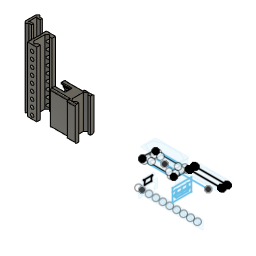
2022_09_14_ThetaSStereoOnPicaTinny v2 (Autodesk Fusion 360 design; units mm, degrees)
Autodesk Fusion 360 part; units mm, degrees
sketch "Sketch1" plane through (0, 0, 0) normal (0, 0, 1) x (1, 0, 0)
  line L0 (9.6991, 0) -> (35.3009, 0)
  line L1 (45, 5.4642) -> (45, 13.4642)
  line L2 (35.2828, 19) -> (9.7172, 19)
  line L3 (0, 13.4642) -> (0, 5.4642)
  line L4 (0, 9.4642) -> (4, 9.4642) construction
  line L5 (4, 9.4642) -> (4, 16.4642) construction
  line L6 (4, 9.4642) -> (4, 2.4642) construction
  line L7 (45, 9.4642) -> (41, 9.4642) construction
  line L8 (41, 9.4642) -> (41, 16.4642) construction
  line L9 (41, 9.4642) -> (41, 2.4642) construction
  line L10 (3.5218, 16.4642) -> (3, 16.4642)
  line L11 (3.3009, 2.4642) -> (3, 2.4642)
  line L12 (41.6991, 2.4642) -> (42, 2.4642)
  line L13 (41.7172, 16.4642) -> (42, 16.4642)
  line L14 (4, 9.4642) -> (9, 9.4642) construction
  line L15 (41, 9.4642) -> (36, 9.4642) construction
  line L16 (36, 9.4642) -> (36, 19) construction
  line L17 (36, 9.4642) -> (36, 0) construction
  line L18 (9, 9.4642) -> (9, 0) construction
  line L19 (9, 9.4642) -> (9, 19) construction
  line L20 (4.4265, 16.6805) -> (8.3603, 18.6756)
  line L21 (36.6397, 18.6756) -> (40.3603, 16.7887)
  line L22 (40.3729, 2.1552) -> (36.6271, 0.3091)
  line L23 (8.3729, 0.3091) -> (4.6271, 2.1552)
  line L24 (0, -1.771) -> (45, -1.771)
  line L25 (47, 0.229) -> (47, 18.6995)
  line L26 (45, 20.6995) -> (0, 20.6995)
  line L27 (-2, 18.6995) -> (-2, 0.229)
  arc A0 (47, 18.6995) -> (45, 20.6995) centre (45, 18.6995) ccw
  arc A1 (45, -1.771) -> (47, 0.229) centre (45, 0.229) ccw
  arc A2 (-2, 0.229) -> (0, -1.771) centre (0, 0.229) ccw
  arc A3 (0, 20.6995) -> (-2, 18.6995) centre (0, 18.6995) ccw
  arc A4 (3.5218, 16.4642) -> (4.4265, 16.6805) centre (3.5218, 18.4642) ccw
  arc A5 (4.6271, 2.1552) -> (3.3009, 2.4642) centre (3.3009, -0.5358) ccw
  arc A6 (40.3603, 16.7887) -> (41.7172, 16.4642) centre (41.7172, 19.4642) ccw
  arc A7 (41.6991, 2.4642) -> (40.3729, 2.1552) centre (41.6991, -0.5358) ccw
  arc A8 (45, 13.4642) -> (42, 16.4642) centre (42, 13.4642) ccw
  arc A9 (42, 2.4642) -> (45, 5.4642) centre (42, 5.4642) ccw
  arc A10 (0, 5.4642) -> (3, 2.4642) centre (3, 5.4642) ccw
  arc A11 (3, 16.4642) -> (0, 13.4642) centre (3, 13.4642) ccw
  arc A12 (9.7172, 19) -> (8.3603, 18.6756) centre (9.7172, 16) ccw
  arc A13 (36.6397, 18.6756) -> (35.2828, 19) centre (35.2828, 16) ccw
  arc A14 (35.3009, 0) -> (36.6271, 0.3091) centre (35.3009, 3) ccw
  arc A15 (8.3729, 0.3091) -> (9.6991, 0) centre (9.6991, 3) ccw
  line L28 (0, 9.4642) -> (-2, 9.4642) construction
  line L29 (45, 9.4642) -> (47, 9.4642) construction
  line L30 (9, 9.4642) -> (36, 9.4642)
  circle A16 centre (22.5, 9.4642) radius 2.5
  line L31 (22.5, 9.4642) -> (85.5, 9.4642)
  circle A17 centre (85.5, 9.4642) radius 2.5
  point P0 (45, 0)
  point P1 (0, 19)
  dimension "d1" = 45
  dimension "d2" = 19
  dimension "d3" = 4
  dimension "d4" = 7
  dimension "d5" = 7
  dimension "d6" = 4
  dimension "d7" = 7
  dimension "d8" = 7
  dimension "d9" = 5
  dimension "d10" = 5
  dimension "d12" = 2
  dimension "d14" = 3
  dimension "d15" = 3
  dimension "d16" = 3
  dimension "d17" = 3
  dimension "d20" = 2
  dimension "d21" = 2
  dimension "d24" = 5
  dimension "d25" = 63
  dimension "d26" = 5
  constraint horizontal L0
  constraint vertical L1
  constraint horizontal L2
  constraint vertical L3
  constraint perpendicular L3 L4
  constraint perpendicular L4 L5
  constraint perpendicular L4 L6
  constraint perpendicular L1 L7
  constraint perpendicular L7 L8
  constraint perpendicular L7 L9
  constraint perpendicular L3 L10
  constraint perpendicular L3 L11
  constraint perpendicular L1 L12
  constraint perpendicular L1 L13
  constraint perpendicular L6 L14
  constraint perpendicular L9 L15
  constraint coincident L2 L16.end
  constraint perpendicular L2 L16
  constraint coincident L0 L17.end
  constraint perpendicular L0 L17
  constraint coincident L0 L18.end
  constraint perpendicular L0 L18
  constraint coincident L2 L19.end
  constraint perpendicular L2 L19
  constraint parallel L0 L24
  constraint parallel L1 L25
  constraint parallel L2 L26
  constraint parallel L3 L27
  constraint tangent L26 A0
  constraint tangent L25 A0
  constraint tangent L25 A1
  constraint tangent L24 A1
  constraint equal A0 A1
  constraint tangent L24 A2
  constraint tangent L27 A2
  constraint equal A0 A2
  constraint tangent L27 A3
  constraint tangent L26 A3
  constraint equal A0 A3
  constraint coincident L5.end L10
  constraint coincident L5.end L20
  constraint tangent L10 A4
  constraint tangent L20 A4
  constraint equal A0 A4
  constraint coincident L6.end L11
  constraint coincident L6.end L23
  constraint tangent L11 A5
  constraint tangent L23 A5
  constraint coincident L8.end L13
  constraint coincident L8.end L21
  constraint tangent L13 A6
  constraint tangent L21 A6
  constraint coincident L9.end L12
  constraint coincident L9.end L22
  constraint tangent L12 A7
  constraint tangent L22 A7
  constraint equal A6 A7
  constraint coincident L1 L7.start
  constraint tangent L13 A8
  constraint tangent L1 A8
  constraint coincident P0 L1
  constraint tangent L1 A9
  constraint tangent L12 A9
  constraint equal A8 A9
  constraint coincident L3 L4.start
  constraint coincident origin L3
  constraint tangent L11 A10
  constraint tangent L3 A10
  constraint equal A8 A10
  constraint coincident P1 L3
  constraint tangent L3 A11
  constraint tangent L10 A11
  constraint equal A8 A11
  constraint coincident L19.end L20
  constraint coincident P1 L2
  constraint tangent L20 A12
  constraint tangent L2 A12
  constraint coincident L16.end L21
  constraint tangent L2 A13
  constraint tangent L21 A13
  constraint equal A12 A13
  constraint coincident L17.end L22
  constraint coincident P0 L0
  constraint tangent L22 A14
  constraint tangent L0 A14
  constraint equal A12 A14
  constraint coincident L18.end L23
  constraint coincident origin L0
  constraint tangent L23 A15
  constraint tangent L0 A15
  constraint equal A12 A15
  constraint midpoint L27 L28.end
  constraint midpoint L25 L29.end
  constraint perpendicular L25 L29
  constraint perpendicular L27 L28
  constraint midpoint L30 A16.centre
  constraint coincident A16.centre L31.start
  constraint parallel L29 L31
  constraint coincident L31.end A17.centre
  measures "d1" distance of origin P0
  measures "d2" distance of origin P1
  measures "d3" distance of L4.start L4.end
  measures "d4" distance of L4.end L5.end
  measures "d5" distance of L4.end L6.end
  measures "d6" distance of L7.start L7.end
  measures "d7" distance of L7.end L8.end
  measures "d8" distance of L7.end L9.end
  measures "d9" distance of L4.end L14.end
  measures "d10" distance of L7.end L15.end
  measures "d12" radius of A0
  measures "d14" radius of A5
  measures "d15" radius of A6
  measures "d16" radius of A8
  measures "d17" radius of A12
  measures "d20" horizontal distance of L7.start L29.end
  measures "d21" distance of L4.start L28.end
  measures "d24" diameter of A16
  measures "d25" distance of A16.centre L31.end
  measures "d26" diameter of A17
extrude "Extrude1" add sketch "Sketch1" along normal blind 15 contours L24 L25 L26 L27 A0 A1 A2 A3 makes body 1
extrude "Extrude2" add sketch "Sketch1" against normal blind 10 contours L0 L1 L2 L3 L10 L11 L12 L13 L20 L21 L22 L23 A4 A5 A6 A7 A8 A9 A10 A11 A12 A13 A14 A15 | L24 L25 L26 L27 A0 A1 A2 A3 | L30 A16 L31 | L30 A16 L31 bodies 1
sketch "Sketch2" plane through (47, 0, 0) normal (1, 0, 0) x (0, 1, 0)
  line L0 (18.6995, -10) -> (18.6995, 15)
  line L1 (18.6995, 15) -> (0.229, 15)
  line L2 (0.229, 15) -> (0.229, -10)
  line L3 (0.229, -10) -> (18.6995, -10)
  line L4 (-0.697, -22.5039) -> (2.068, -25.5039)
  line L5 (2.8515, -21.5039) -> (2.8515, -22.5039)
  line L6 (9.903, -22.5039) -> (9.903, -21.5039)
  line L7 (17.738, -25.5039) -> (2.068, -25.5039)
  line L8 (2.068, -19.9555) -> (2.068, -16.1839)
  line L9 (9.903, -25.5039) -> (9.903, -22.5039)
  line L10 (9.903, -21.5039) -> (2.8515, -21.5039)
  line L11 (16.9545, -21.5039) -> (16.9545, -22.5039)
  line L12 (9.903, -22.5039) -> (20.503, -22.5039)
  line L13 (17.738, -25.5039) -> (20.503, -22.5039)
  line L14 (9.903, -21.5039) -> (16.9545, -21.5039)
  line L15 (20.503, -22.5039) -> (17.738, -19.9555)
  line L16 (9.903, -22.5039) -> (-0.697, -22.5039)
  line L17 (-0.697, -22.5039) -> (2.068, -19.9555)
  line L18 (2.068, -16.1839) -> (17.738, -16.1839)
  line L19 (-3.7288, -11.1839) -> (23.503, -11.1839)
  line L20 (23.503, -11.1839) -> (23.503, -29.4392)
  line L21 (23.503, -29.4392) -> (-3.7288, -29.4392)
  line L22 (-3.7288, -29.4392) -> (-3.7288, -11.1839)
  line L23 (20.503, -22.5039) -> (23.503, -22.5039) construction
  line L24 (20.503, -22.5039) -> (-0.697, -22.5039)
  line L25 (9.903, -21.5039) -> (9.903, -16.1839)
  line L26 (2.068, -16.1839) -> (-3.7288, -16.1839)
  line L27 (17.738, -16.1839) -> (23.503, -16.1839)
  line L28 (17.738, -16.1839) -> (17.738, -19.9555)
  line L29 (18.338, -16.1839) -> (18.338, -19.6926)
  line L30 (21.3508, -22.4694) -> (18.338, -19.6926)
  line L31 (18.0009, -26.1039) -> (21.3508, -22.4694)
  line L32 (18.0009, -26.1039) -> (1.805, -26.1039)
  line L33 (-1.5449, -22.4694) -> (1.805, -26.1039)
  line L34 (-1.5449, -22.4694) -> (1.468, -19.6926)
  line L35 (1.468, -19.6926) -> (1.468, -16.1839)
  circle A0 centre (9.903, -22.5039) radius 0.05
  dimension "d27" = 3
  dimension "d30" = -0.6
  dimension "d41" = 0.1
  constraint horizontal L19
  constraint vertical L20
  constraint horizontal L21
  constraint vertical L22
  constraint parallel L12 L23
  constraint parallel L16 L24
  constraint coincident L20 L23.end
  constraint midpoint L18 L25.end
  constraint perpendicular L18 L25
  constraint perpendicular L18 L28
  constraint perpendicular L8 L18
  constraint perpendicular L7 L8
  constraint coincident L22 L26.end
  constraint perpendicular L22 L26
  constraint coincident L20 L27.end
  constraint perpendicular L20 L27
  constraint coincident L6.start L9.end
  measures "d27" distance of L12.end L23.end
  measures "d41" diameter of A0
extrude "Extrude3" add sketch "Sketch2" along normal blind -49 and the other way blind -65 separate body contours L20 L21 L22 L26 L27 L29 L30 L31 L32 L33 L34 L35 makes body 2
copy_body "CopyPasteBodies1" bodies 1 makes body 3
move_body "Move1" bodies 3 to x (1, 0, 0) y (0, 1, 0) z (0, 0, 1) at (63, 0, 0)
extrude "Extrude4" cut 1 faces at (112, -1.1562, -26.0042) along direction (-1, 0, 0) blind 2 on bodies 2 bodies 2
extrude "Extrude5" add sketch "Sketch2" along normal blind 63 and the other way blind 49 separate body contours L4 L7 L9 L16 L24 A0 | L5 L8 L10 L16 L17 L18 L24 L25 | L5 L6 L10 L16 L24 A0 | L7 L9 L12 L13 L24 A0 | L6 L16 L24 A0 | L9 L16 L24 A0 | L9 L12 L24 A0 | L6 L11 L12 L14 L24 A0 | L11 L12 L14 L15 L18 L24 L25 L28 | L6 L12 L24 A0 makes body 4
move_body "Move2" bodies 2 4 to x (1, 0, 0) y (0, -1, 0) z (0, 0, -1) at (0, 19.8059, -45.0079)
move_body "Move3" bodies 2 to x (1, 0, 0) y (0, 1, 0) z (0, 0, 1) at (0, -0.4546, 5.5686)
extrude "Extrude6" cut 1 faces at (-2, 20.5075, -13.4351) along direction (1, 0, 0) blind 63 on bodies 2 bodies 2
combine "Combine1" operation add target body 2 tool bodies 3
extrude "Extrude7" add sketch "Sketch2" along normal blind -30 and the other way blind -45 separate body contours L20 L21 L22 L26 L27 L29 L30 L31 L32 L33 L34 L35 makes body 5
move_body "Move4" bodies 5 to x (-1, 0, 0) y (0, 1, 0) z (0, 0, -1) at (184, 0, -58.8785)
move_body "Move5" bodies 5 to x (1, 0, 0) y (0, 1, 0) z (0, 0, 1) at (-75.5, 0.0159, 0.6153)
extrude "Extrude8" add 1 faces at (16.5, -1.1403, -32.259) along direction (-1, 0, 0) blind 20 on bodies 5 bodies 5 4
extrude "Extrude9" cut 1 faces at (-3.5, -1.1403, -32.259) along direction (1, 0, 0) blind 1.5 on bodies 5 bodies 5
sketch "Sketch3" plane through (0, -3.7129, 0) normal (0, -1, 0) x (1, 0, 0)
  line L0 (-2, -28.8239) -> (-2, -42.0792)
  line L1 (-2, -42.0792) -> (91.5, -42.0792)
  line L2 (91.5, -42.0792) -> (91.5, -28.8239)
  line L3 (91.5, -28.8239) -> (-2, -28.8239)
sketch "Sketch4" plane through (0, -3.7129, 0) normal (0, -1, 0) x (1, 0, 0)
  line L0 (-2, -35.5) -> (3, -35.5)
  circle A0 centre (3, -35.5) radius 2.5
  circle A1 centre (13, -35.5) radius 2.5
  circle A2 centre (23, -35.5) radius 2.5
  circle A3 centre (33, -35.5) radius 2.5
  circle A4 centre (43, -35.5) radius 2.5
  circle A5 centre (53, -35.5) radius 2.5
  circle A6 centre (63, -35.5) radius 2.5
  circle A7 centre (73, -35.5) radius 2.5
  circle A8 centre (83, -35.5) radius 2.5
  dimension "d54" = 5
  dimension "d55" = 5
  dimension "d58" = 10
  dimension "d59" = 0
  constraint horizontal L0
  constraint coincident L0.end A0.centre
  measures "d54" distance of L0.start L0.end
  measures "d55" diameter of A0
extrude "Extrude10" cut sketch "Sketch4" against normal blind 39 bodies 5
move_body "Move6" bodies 5 to x (1, 0, 0) y (0, 1, 0) z (0, 0, 1) at (0, 0, -7)
sketch "Sketch5" plane through (-2, 0, 0) normal (-1, 0, 0) x (0, -1, 0)
  line L0 (-17.738, -26.5039) -> (-20.503, -29.5039)
  line L1 (-20.503, -29.5039) -> (-17.738, -32.0523)
  line L2 (-17.738, -32.0523) -> (-17.738, -35.8239)
  line L3 (-17.738, -35.8239) -> (-23.5188, -35.8239)
  line L4 (-23.5188, -35.8239) -> (-23.5188, -49.0792)
  line L5 (-23.5188, -49.0792) -> (-18.3538, -49.0792)
  line L6 (-18.3538, -49.0792) -> (-18.3538, -45.5706)
  line L7 (-18.3538, -45.5706) -> (-21.3667, -42.7938)
  line L8 (-21.3667, -42.7938) -> (-18.0168, -39.1592)
  line L9 (-18.0168, -39.1592) -> (-1.8209, -39.1592)
  line L10 (-1.8209, -39.1592) -> (1.529, -42.7938)
  line L11 (1.529, -42.7938) -> (-1.4838, -45.5706)
  line L12 (-1.4838, -45.5706) -> (-1.4838, -49.0792)
  line L13 (-1.4838, -49.0792) -> (3.7129, -49.0792)
  line L14 (3.7129, -49.0792) -> (3.7129, -35.8239)
  line L15 (3.7129, -35.8239) -> (-2.068, -35.8239)
  line L16 (-2.068, -35.8239) -> (-2.068, -32.0523)
  line L17 (-2.068, -32.0523) -> (0.697, -29.5039)
  line L18 (0.697, -29.5039) -> (-2.068, -26.5039)
  line L19 (-2.068, -26.5039) -> (-17.738, -26.5039)
  line L20 (-3.7296, -29.5039) -> (-16.0764, -29.5039)
  line L21 (-16.0764, -29.5039) -> (-14.738, -30.7375)
  line L22 (-14.738, -30.7375) -> (-14.738, -36.1592)
  line L23 (-14.738, -36.1592) -> (-5.068, -36.1592)
  line L24 (-5.068, -36.1592) -> (-5.068, -30.7375)
  line L25 (-5.068, -30.7375) -> (-3.7296, -29.5039)
  dimension "d65" = -3
extrude "Extrude11" cut sketch "Sketch5" against normal blind 145 contours L20 L21 L22 L23 L24 L25 bodies 5
sketch "Sketch6" plane through (0, 0, 15) normal (0, 0, 1) x (-1, 0, 0)
  line L0 (-8.3729, -0.3091) -> (-4.6271, -2.1552)
  arc A0 (-4.6271, -2.1552) -> (-3.3009, -2.4642) centre (-3.3009, 0.5358) ccw
  line L1 (-3.3009, -2.4642) -> (-3, -2.4642)
  arc A1 (0, -5.4642) -> (-3, -2.4642) centre (-3, -5.4642) ccw
  line L2 (0, -5.4642) -> (0, -13.4642)
  arc A2 (-3, -16.4642) -> (0, -13.4642) centre (-3, -13.4642) ccw
  line L3 (-3, -16.4642) -> (-3.5218, -16.4642)
  arc A3 (-3.5218, -16.4642) -> (-4.4265, -16.6805) centre (-3.5218, -18.4642) ccw
  line L4 (-4.4265, -16.6805) -> (-8.3603, -18.6756)
  arc A4 (-9.7172, -19) -> (-8.3603, -18.6756) centre (-9.7172, -16) ccw
  line L5 (-9.7172, -19) -> (-35.2828, -19)
  arc A5 (-36.6397, -18.6756) -> (-35.2828, -19) centre (-35.2828, -16) ccw
  line L6 (-36.6397, -18.6756) -> (-40.3603, -16.7887)
  arc A6 (-40.3603, -16.7887) -> (-41.7172, -16.4642) centre (-41.7172, -19.4642) ccw
  line L7 (-41.7172, -16.4642) -> (-42, -16.4642)
  arc A7 (-45, -13.4642) -> (-42, -16.4642) centre (-42, -13.4642) ccw
  line L8 (-45, -13.4642) -> (-45, -5.4642)
  arc A8 (-42, -2.4642) -> (-45, -5.4642) centre (-42, -5.4642) ccw
  line L9 (-42, -2.4642) -> (-41.6991, -2.4642)
  arc A9 (-41.6991, -2.4642) -> (-40.3729, -2.1552) centre (-41.6991, 0.5358) ccw
  line L10 (-40.3729, -2.1552) -> (-36.6271, -0.3091)
  arc A10 (-35.3009, 0) -> (-36.6271, -0.3091) centre (-35.3009, -3) ccw
  line L11 (-35.3009, 0) -> (-9.6991, 0)
  arc A11 (-8.3729, -0.3091) -> (-9.6991, 0) centre (-9.6991, -3) ccw
  arc A12 (0, -20.6995) -> (2, -18.6995) centre (0, -18.6995) ccw
  line L12 (2, -18.6995) -> (2, -0.229)
  arc A13 (2, -0.229) -> (0, 1.771) centre (0, -0.229) ccw
  line L13 (0, 1.771) -> (-45, 1.771)
  arc A14 (-45, 1.771) -> (-47, -0.229) centre (-45, -0.229) ccw
  line L14 (-47, -0.229) -> (-47, -18.6995)
  arc A15 (-47, -18.6995) -> (-45, -20.6995) centre (-45, -18.6995) ccw
  line L15 (-45, -20.6995) -> (0, -20.6995)
sketch "Sketch7" plane through (0, 0, 15) normal (0, 0, 1) x (-1, 0, 0)
  line L0 (-71.3729, -0.3091) -> (-67.6271, -2.1552)
  arc A0 (-67.6271, -2.1552) -> (-66.3009, -2.4642) centre (-66.3009, 0.5358) ccw
  line L1 (-66.3009, -2.4642) -> (-66, -2.4642)
  arc A1 (-63, -5.4642) -> (-66, -2.4642) centre (-66, -5.4642) ccw
  line L2 (-63, -5.4642) -> (-63, -13.4642)
  arc A2 (-66, -16.4642) -> (-63, -13.4642) centre (-66, -13.4642) ccw
  line L3 (-66, -16.4642) -> (-66.5218, -16.4642)
  arc A3 (-66.5218, -16.4642) -> (-67.4265, -16.6805) centre (-66.5218, -18.4642) ccw
  line L4 (-67.4265, -16.6805) -> (-71.3603, -18.6756)
  arc A4 (-72.7172, -19) -> (-71.3603, -18.6756) centre (-72.7172, -16) ccw
  line L5 (-72.7172, -19) -> (-98.2828, -19)
  arc A5 (-99.6397, -18.6756) -> (-98.2828, -19) centre (-98.2828, -16) ccw
  line L6 (-99.6397, -18.6756) -> (-103.3603, -16.7887)
  arc A6 (-103.3603, -16.7887) -> (-104.7172, -16.4642) centre (-104.7172, -19.4642) ccw
  line L7 (-104.7172, -16.4642) -> (-105, -16.4642)
  arc A7 (-108, -13.4642) -> (-105, -16.4642) centre (-105, -13.4642) ccw
  line L8 (-108, -13.4642) -> (-108, -5.4642)
  arc A8 (-105, -2.4642) -> (-108, -5.4642) centre (-105, -5.4642) ccw
  line L9 (-105, -2.4642) -> (-104.6991, -2.4642)
  arc A9 (-104.6991, -2.4642) -> (-103.3729, -2.1552) centre (-104.6991, 0.5358) ccw
  line L10 (-103.3729, -2.1552) -> (-99.6271, -0.3091)
  arc A10 (-98.3009, 0) -> (-99.6271, -0.3091) centre (-98.3009, -3) ccw
  line L11 (-98.3009, 0) -> (-72.6991, 0)
  arc A11 (-71.3729, -0.3091) -> (-72.6991, 0) centre (-72.6991, -3) ccw
  arc A12 (-63, -20.6995) -> (-61, -18.6995) centre (-63, -18.6995) ccw
  line L12 (-61, -18.6995) -> (-61, -0.229)
  arc A13 (-61, -0.229) -> (-63, 1.771) centre (-63, -0.229) ccw
  line L13 (-63, 1.771) -> (-108, 1.771)
  arc A14 (-108, 1.771) -> (-110, -0.229) centre (-108, -0.229) ccw
  line L14 (-110, -0.229) -> (-110, -18.6995)
  arc A15 (-110, -18.6995) -> (-108, -20.6995) centre (-108, -18.6995) ccw
  line L15 (-108, -20.6995) -> (-63, -20.6995)
  line L16 (-108, -5.4642) -> (-63, -5.4642)
  line L17 (-61, -5.4642) -> (-61, -13.4642)
  line L18 (-61, -13.4642) -> (-63, -13.4642)
  line L19 (-108, -13.4642) -> (-63, -13.4642)
  line L20 (-108, -13.4642) -> (-110, -13.4642)
  line L21 (-108, -5.4642) -> (-110, -5.4642)
  line L22 (-63, -5.4642) -> (-61, -5.4642)
  constraint coincident L8.end A8.end
  constraint coincident A1.start L2.start
  constraint coincident L12 L17.start
  constraint coincident L12 L17.end
  constraint perpendicular L16 L17
  constraint coincident L2.end A2.end
  constraint coincident A7.start L8.start
  constraint coincident L14 L20.end
  constraint perpendicular L14 L20
  constraint coincident L14 L21.end
  constraint perpendicular L14 L21
  constraint perpendicular L17 L22
  constraint parallel L18 L19
extrude "Extrude12" cut sketch "Sketch7" against normal blind 15 contours L8 L14 L20 L21 bodies 2
fillet "Fillet1" radius 1 4 edges at (108, 5.4642, 7.5) (110, 5.4642, 7.5) (110, 13.4642, 7.5) (108, 13.4642, 7.5) on bodies 2
fillet "Fillet2" radius 2 9 edges at (110, -4.1516, -16.6277) (110, -1.9613, -10) (85.5, -4.1516, -10) (110, 20.8898, -10) (110, 23.0801, -16.6277) (85.5, 23.0801, -10) (61, -4.1516, -16.6277) (61, 23.0801, -16.6277) (61, 20.8898, -10) on bodies 2
copy_body "CopyPasteBodies2" bodies 5 2 makes body 6 makes body 7
move_body "Move7" bodies 6 7 to x (0, 0, 1) y (0, 1, 0) z (-1, 0, 0) at (-28.5039, 0, -24.5039)
move_body "Move8" bodies 7 to x (1, 0, 0) y (0, 1, 0) z (0, 0, 1) at (41.5039, 0.4387, -63)
move_body "Move9" bodies 6 7 to x (1, 0, 0) y (0, 1, 0) z (0, 0, 1) at (-170, 0, 0)
move_body "Move10" bodies 7 to x (1, 0, 0) y (0, 1, 0) z (0, 0, 1) at (40, 0, 0)
hidden bodies 1 2 5
